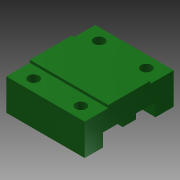
# Autodesk Inventor part: Linear Bearing Platform Adapter
Saved by Autodesk Inventor 2015 SP1 (Build 190203100, 203)
## iProperties
Created: 2015-03-04
Part Number: Linear Bearing Platform Adapter
Material: PC/ABS Plastic
Document SubType Name: Modeling
Designer: Andrew
Density: 0.357273 g/cm^3
Appearance: Smooth - Dark Forest Green
Author: Andrew
Autodesk Inventor part; units mm, degrees
ref_plane "YZ Plane" through (0, 0, 0) normal (1, 0, 0) x (0, 1, 0)
ref_plane "XZ Plane" through (0, 0, 0) normal (0, 1, 0) x (-1, 0, 0)
ref_plane "XY Plane" through (0, 0, 0) normal (0, 0, 1) x (1, 0, 0)
sketch "Sketch1" plane through (0, 0, 0) normal (0, 0, 1) x (1, 0, 0)
  line L0 (-15, -17) -> (15, -17)
  line L1 (15, -17) -> (15, 17)
  line L2 (15, 17) -> (-15, 17)
  line L3 (-15, 17) -> (-15, -17)
  line L4 (-15, -17) -> (15, 17) construction
  line L5 (15, -17) -> (-15, 17) construction
  line L6 (-15, -8) -> (15, -8)
  line L7 (15, -8) -> (15, 8)
  line L8 (15, 8) -> (-15, 8)
  line L9 (-15, 8) -> (-15, -8)
  line L10 (-15, -8) -> (15, 8) construction
  line L11 (15, -8) -> (-15, 8) construction
  circle A0 centre (-9, 12.5) radius 2 construction
  point P0 (0, 0)
  dimension "d0" = 34
  dimension "d1" = 30
  dimension "d2" = 16
  dimension "d3" = 4
  dimension "d4" = 6
  dimension "d5" = 4.5
  constraints: 24 end point, 4 midpoint, 4 parallel, 2 horizontal, 2 perpendicular, 1 centre point, 1 coincident, 1 point on line
  measures "d0" distance of L0.end L1.end
  measures "d1" distance of L1.end L2.end
  measures "d2" distance between parallel lines of L6 L8
  measures "d3" diameter of A0
  measures "d4" distance from line of L3 A0.centre
  measures "d5" distance from line of L2 A0.centre
extrude "Extrusion1" add sketch "Sketch1" along normal blind 2 contours L3 L6 L1 L0 | L3 L2 L1 L8
extrude "Extrusion2" add sketch "Sketch1" along normal blind 3 contours L3 L8 L1 L6
hole "Hole1" at (-9, 12.5, 0) direction (0, 0, 1) diameter 4 end through all
pattern_linear "Rectangular Pattern1" count 2 spacing 18 along (1, 0, 0) count 2 spacing 25 along (0, -1, 0) of "Hole1"
sketch "Sketch2" plane through (0, 0, 0) normal (0, 0, -1) x (-1, 0, 0)
  circle A0 centre (-9, -12.5) radius 2 projected
  circle A1 centre (9, -12.5) radius 2 projected
  circle A2 centre (-9, 12.5) radius 2 projected
  circle A3 centre (9, 12.5) radius 2 projected
  line L0 (-15, -17) -> (-15, 17) projected
  line L1 (15, -17) -> (-15, -17) projected
  line L2 (15, 17) -> (15, -17) projected
  line L3 (-15, 17) -> (15, 17) projected
  point P0 (0, 0)
extrude "Extrusion3" add sketch "Sketch2" along normal blind 5
sketch "Sketch3" plane through (0, 0, -5) normal (0, 0, -1) x (-1, 0, 0)
  circle A0 centre (9, 12.5) radius 2 projected
  circle A1 centre (-9, 12.5) radius 2 projected
  circle A2 centre (9, -12.5) radius 2 projected
  circle A3 centre (-9, -12.5) radius 2 projected
  line L0 (-15, 17) -> (-15, -17) projected
  line L1 (-15, -17) -> (15, -17) projected
  line L2 (15, -17) -> (15, 17) projected
  line L3 (15, 17) -> (-15, 17) projected
  line L4 (15, -2.5) -> (-15, -2.5)
  line L5 (-15, -2.5) -> (-15, 2.5)
  line L6 (-15, 2.5) -> (15, 2.5)
  line L7 (15, 2.5) -> (15, -2.5)
  line L8 (15, -2.5) -> (-15, 2.5) construction
  line L9 (-15, -2.5) -> (15, 2.5) construction
  line L10 (15, 10) -> (-15, 10)
  line L11 (-15, 10) -> (-15, -10)
  line L12 (-15, -10) -> (15, -10)
  line L13 (15, -10) -> (15, 10)
  line L14 (15, 10) -> (-15, -10) construction
  line L15 (-15, 10) -> (15, -10) construction
  point P0 (0, 0)
  dimension "d25" = 5
  dimension "d28" = 20
  constraints: 24 end point, 4 midpoint, 4 parallel, 2 horizontal, 2 perpendicular, 2 point on line
  measures "d25" distance between parallel lines of L4 L6
  measures "d28" distance between parallel lines of L10 L12
extrude "Extrusion4" add sketch "Sketch3" along normal blind 2 contours L6 L2 L4 L0
extrude "Extrusion5" add sketch "Sketch3" along normal blind 5 contours L3 L2 L10 L0 | L12 L2 L1 L0
body "Solid1"
